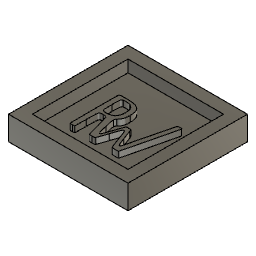
Experiment-Initials Revisited v3 (Autodesk Fusion 360 design; units mm, degrees)
Autodesk Fusion 360 part; units mm, degrees
sketch "Sketch2" plane through (0, 0, 0) normal (0, 0, 1) x (1, 0, 0)
  line L0 (0, 0) -> (100, 0)
  line L1 (100, 0) -> (100, 100)
  line L2 (100, 100) -> (0, 100)
  line L3 (0, 100) -> (0, 0)
  constraint horizontal L0
  constraint vertical L1
  constraint horizontal L2
  constraint vertical L3
  constraint coincident L0.start L3.end
extrude "Extrude3" add sketch "Sketch2" along normal blind 20
sketch "Sketch3" plane through (0, 0, 20) normal (0, 0, 1) x (-1, 0, 0)
  line L0 (0, -100) -> (0, 0)
  line L1 (0, 0) -> (-100, 0)
  line L2 (-100, 0) -> (-100, -100)
  line L3 (-100, -100) -> (0, -100)
  line L4 (-10, -10) -> (-90, -10)
  line L5 (-90, -10) -> (-90, -90)
  line L6 (-90, -90) -> (-10, -90)
  line L7 (-10, -90) -> (-10, -10)
  constraint horizontal L4
  constraint vertical L5
  constraint horizontal L6
  constraint vertical L7
extrude "Extrude4" cut sketch "Sketch3" against normal blind 10 contours L4 L5 L6 L7
sketch "Sketch4" plane through (0, 0, 10) normal (0, 0, 1) x (-1, 0, 0)
  line L0 (-10, -90) -> (-10, -10)
  line L1 (-10, -10) -> (-90, -10)
  line L2 (-90, -10) -> (-90, -90)
  line L3 (-90, -90) -> (-10, -90)
  spline S0 degree 3 poles (-75.4628, -68.295) (-73.8753, -68.1891) (-73.6636, -68.1362) (-73.5313, -67.6071) knots 0 0 0 0 1 1 1 1
  spline S1 degree 3 poles (-73.5313, -67.6071) (-72.473, -63.0562) (-68.3455, -46.4404) (-68.1338, -45.8583) knots 0 0 0 0 1 1 1 1
  spline S2 degree 3 poles (-68.1338, -45.8583) (-67.7369, -44.7471) (-64.7736, -31.8618) (-64.5355, -30.3008) knots 0 0 0 0 1 1 1 1
  spline S3 degree 3 poles (-64.5355, -30.3008) (-64.3503, -28.8456) (-64.0063, -28.8456) (-63.8211, -30.3273) knots 0 0 0 0 1 1 1 1
  spline S4 degree 3 poles (-63.8211, -30.3273) (-63.7417, -30.8829) (-62.4453, -34.6929) (-60.9371, -38.7939) knots 0 0 0 0 1 1 1 1
  line L4 (-60.9371, -38.7939) -> (-58.1855, -46.2552)
  line L5 (-58.1855, -46.2552) -> (-55.4073, -46.2552)
  line L6 (-55.4073, -46.2552) -> (-52.6028, -46.2552)
  line L7 (-52.6028, -46.2552) -> (-50.0363, -38.4764)
  spline S5 degree 3 poles (-50.0363, -38.4764) (-48.634, -34.2166) (-47.4698, -30.4596) (-47.4698, -30.1421) knots 0 0 0 0 1 1 1 1
  spline S6 degree 3 poles (-47.4698, -30.1421) (-47.4698, -29.0308) (-46.9936, -29.6129) (-46.8348, -30.9887) knots 0 0 0 0 1 1 1 1
  spline S7 degree 3 poles (-46.8348, -30.9887) (-46.729, -31.7296) (-45.9882, -35.275) (-45.1944, -38.8204) knots 0 0 0 0 1 1 1 1
  line L8 (-45.1944, -38.8204) -> (-43.7657, -45.2762)
  line L9 (-43.7657, -45.2762) -> (-44.824, -46.1758)
  spline S8 degree 3 poles (-44.824, -46.1758) (-46.3057, -47.4723) (-47.1523, -49.0333) (-47.6021, -51.4146) knots 0 0 0 0 1 1 1 1
  spline S9 degree 3 poles (-47.6021, -51.4146) (-48.0784, -53.7958) (-48.1048, -55.8066) (-47.708, -58.1614) knots 0 0 0 0 1 1 1 1
  spline S10 degree 3 poles (-47.708, -58.1614) (-47.1788, -61.5216) (-45.7765, -63.6648) (-43.263, -65.0141) knots 0 0 0 0 1 1 1 1
  spline S11 degree 3 poles (-43.263, -65.0141) (-40.8288, -66.3106) (-38.5269, -66.6281) (-31.833, -66.6281) knots 0 0 0 0 1 1 1 1
  line L10 (-31.833, -66.6281) -> (-26.0386, -66.6281)
  line L11 (-26.0386, -66.6281) -> (-26.0386, -44.8)
  line L12 (-26.0386, -44.8) -> (-26.0386, -22.9718)
  line L13 (-26.0386, -22.9718) -> (-29.2136, -22.9718)
  line L14 (-29.2136, -22.9718) -> (-32.3886, -22.9718)
  line L15 (-32.3886, -22.9718) -> (-32.3886, -33.2377)
  line L16 (-32.3886, -33.2377) -> (-32.3886, -43.4771)
  line L17 (-32.3886, -43.4771) -> (-34.6905, -43.4241)
  line L18 (-34.6905, -43.4241) -> (-36.9659, -43.3712)
  line L19 (-36.9659, -43.3712) -> (-39.7969, -33.2377)
  line L20 (-39.7969, -33.2377) -> (-42.6015, -23.1041)
  line L21 (-42.6015, -23.1041) -> (-45.803, -23.0248)
  line L22 (-45.803, -23.0248) -> (-48.978, -22.9454)
  line L23 (-48.978, -22.9454) -> (-51.6503, -30.83)
  spline S12 degree 3 poles (-51.6503, -30.83) (-53.1319, -35.1691) (-54.4019, -39.085) (-54.5078, -39.5083) knots 0 0 0 0 1 1 1 1
  spline S13 degree 3 poles (-54.5078, -39.5083) (-54.8517, -41.1752) (-54.9311, -41.3339) (-55.1692, -40.9371) knots 0 0 0 0 1 1 1 1
  spline S14 degree 3 poles (-55.1692, -40.9371) (-55.3015, -40.7254) (-55.4073, -40.355) (-55.4073, -40.0904) knots 0 0 0 0 1 1 1 1
  spline S15 degree 3 poles (-55.4073, -40.0904) (-55.4073, -39.8258) (-56.8096, -35.8835) (-58.503, -31.3062) knots 0 0 0 0 1 1 1 1
  line L24 (-58.503, -31.3062) -> (-61.5986, -22.9983)
  line L25 (-61.5986, -22.9983) -> (-65.144, -22.9189)
  spline S16 degree 3 poles (-65.144, -22.9189) (-67.1019, -22.866) (-68.7159, -22.8925) (-68.7688, -22.9718) knots 0 0 0 0 1 1 1 1
  spline S17 degree 3 poles (-68.7688, -22.9718) (-68.8482, -23.1306) (-79.749, -68.1098) (-79.749, -68.3214) knots 0 0 0 0 1 1 1 1
  spline S18 degree 3 poles (-79.749, -68.3214) (-79.749, -68.4802) (-79.0346, -68.4802) (-75.4628, -68.295) knots 0 0 0 0 1 1 1 1
  spline S19 degree 3 poles (-78.1615, -66.6546) (-78.1615, -66.0989) (-68.1603, -24.6123) (-67.9486, -24.2683) knots 0 0 0 0 1 1 1 1
  spline S20 degree 3 poles (-67.9486, -24.2683) (-67.7105, -23.8714) (-62.6569, -23.9773) (-62.3394, -24.3741) knots 0 0 0 0 1 1 1 1
  spline S21 degree 3 poles (-62.3394, -24.3741) (-62.1807, -24.5329) (-60.8048, -28.1577) (-59.2438, -32.3646) knots 0 0 0 0 1 1 1 1
  spline S22 degree 3 poles (-59.2438, -32.3646) (-56.1217, -40.8841) (-55.9894, -41.1752) (-55.3544, -41.5985) knots 0 0 0 0 1 1 1 1
  spline S23 degree 3 poles (-55.3544, -41.5985) (-54.4548, -42.1541) (-53.8992, -40.9635) (-51.3063, -33.026) knots 0 0 0 0 1 1 1 1
  spline S24 degree 3 poles (-51.3063, -33.026) (-49.904, -28.7398) (-48.5811, -24.9562) (-48.3694, -24.6123) knots 0 0 0 0 1 1 1 1
  spline S25 degree 3 poles (-48.3694, -24.6123) (-48.0255, -24.0831) (-47.7873, -24.0302) (-45.7765, -24.0302) knots 0 0 0 0 1 1 1 1
  spline S26 degree 3 poles (-45.7765, -24.0302) (-43.6069, -24.0302) (-43.554, -24.0566) (-43.2894, -24.7446) knots 0 0 0 0 1 1 1 1
  spline S27 degree 3 poles (-43.2894, -24.7446) (-43.1307, -25.1679) (-41.8871, -29.4541) (-40.5642, -34.3225) knots 0 0 0 0 1 1 1 1
  spline S28 degree 3 poles (-40.5642, -34.3225) (-39.1884, -39.2702) (-37.8919, -43.4241) (-37.6009, -43.7681) knots 0 0 0 0 1 1 1 1
  spline S29 degree 3 poles (-37.6009, -43.7681) (-37.1511, -44.3502) (-36.913, -44.4031) (-34.7963, -44.4031) knots 0 0 0 0 1 1 1 1
  spline S30 degree 3 poles (-34.7963, -44.4031) (-31.2244, -44.4031) (-31.489, -45.1968) (-31.3303, -33.7139) knots 0 0 0 0 1 1 1 1
  line L26 (-31.3303, -33.7139) -> (-31.198, -24.1625)
  line L27 (-31.198, -24.1625) -> (-29.3723, -24.0831)
  spline S31 degree 3 poles (-29.3723, -24.0831) (-28.0759, -24.0302) (-27.4673, -24.1096) (-27.3351, -24.3477) knots 0 0 0 0 1 1 1 1
  spline S32 degree 3 poles (-27.3351, -24.3477) (-27.0705, -24.7446) (-27.0176, -64.5114) (-27.2557, -65.1464) knots 0 0 0 0 1 1 1 1
  spline S33 degree 3 poles (-27.2557, -65.1464) (-27.4938, -65.755) (-36.5426, -65.755) (-39.4794, -65.1464) knots 0 0 0 0 1 1 1 1
  spline S34 degree 3 poles (-39.4794, -65.1464) (-44.7976, -64.0616) (-46.8084, -61.2835) (-46.8084, -54.9864) knots 0 0 0 0 1 1 1 1
  spline S35 degree 3 poles (-46.8084, -54.9864) (-46.7819, -50.7531) (-46.2263, -49.1391) (-43.9244, -46.705) knots 0 0 0 0 1 1 1 1
  spline S36 degree 3 poles (-43.9244, -46.705) (-43.2365, -45.9641) (-42.9719, -45.4614) (-42.9719, -44.8529) knots 0 0 0 0 1 1 1 1
  spline S37 degree 3 poles (-42.9719, -44.8529) (-42.9719, -44.3766) (-43.6598, -40.8841) (-44.533, -37.0477) knots 0 0 0 0 1 1 1 1
  spline S38 degree 3 poles (-44.533, -37.0477) (-45.7236, -31.6502) (-46.1998, -29.9568) (-46.6232, -29.5071) knots 0 0 0 0 1 1 1 1
  spline S39 degree 3 poles (-46.6232, -29.5071) (-47.1788, -28.9779) (-47.2053, -28.9779) (-47.708, -29.4277) knots 0 0 0 0 1 1 1 1
  spline S40 degree 3 poles (-47.708, -29.4277) (-48.0519, -29.7187) (-49.0573, -32.391) (-50.4067, -36.4391) knots 0 0 0 0 1 1 1 1
  spline S41 degree 3 poles (-50.4067, -36.4391) (-51.5973, -40.011) (-52.788, -43.4506) (-53.0526, -44.0856) knots 0 0 0 0 1 1 1 1
  line L28 (-53.0526, -44.0856) -> (-53.5553, -45.2233)
  line L29 (-53.5553, -45.2233) -> (-55.4603, -45.1439)
  line L30 (-55.4603, -45.1439) -> (-57.3917, -45.0646)
  line L31 (-57.3917, -45.0646) -> (-58.0267, -43.4771)
  spline S42 degree 3 poles (-58.0267, -43.4771) (-58.3707, -42.6039) (-59.6936, -39.0321) (-60.9901, -35.5396) knots 0 0 0 0 1 1 1 1
  spline S43 degree 3 poles (-60.9901, -35.5396) (-62.2865, -32.0471) (-63.5301, -29.0308) (-63.7946, -28.8721) knots 0 0 0 0 1 1 1 1
  spline S44 degree 3 poles (-63.7946, -28.8721) (-64.1386, -28.581) (-64.3238, -28.6075) (-64.7207, -28.9779) knots 0 0 0 0 1 1 1 1
  spline S45 degree 3 poles (-64.7207, -28.9779) (-65.2763, -29.4806) (-65.3821, -29.851) (-66.6521, -35.275) knots 0 0 0 0 1 1 1 1
  spline S46 degree 3 poles (-66.6521, -35.275) (-67.6311, -39.5348) (-68.6894, -43.7946) (-69.9594, -48.6364) knots 0 0 0 0 1 1 1 1
  spline S47 degree 3 poles (-69.9594, -48.6364) (-70.3828, -50.3033) (-71.5205, -54.96) (-72.4994, -58.9552) knots 0 0 0 0 1 1 1 1
  spline S48 degree 3 poles (-72.4994, -58.9552) (-73.4519, -62.9504) (-74.3515, -66.4429) (-74.4838, -66.7075) knots 0 0 0 0 1 1 1 1
  spline S49 degree 3 poles (-74.4838, -66.7075) (-74.6955, -67.0514) (-75.0923, -67.1573) (-76.4417, -67.1573) knots 0 0 0 0 1 1 1 1
  spline S50 degree 3 poles (-76.4417, -67.1573) (-77.9498, -67.1573) (-78.1615, -67.1043) (-78.1615, -66.6546) knots 0 0 0 0 1 1 1 1
  spline S51 degree 3 poles (-32.759, -63.215) (-31.4096, -62.6329) (-31.3303, -62.236) (-31.3303, -55.1981) knots 0 0 0 0 1 1 1 1
  spline S52 degree 3 poles (-31.3303, -55.1981) (-31.3303, -50.9648) (-31.4361, -48.4248) (-31.6213, -48.0279) knots 0 0 0 0 1 1 1 1
  spline S53 degree 3 poles (-31.6213, -48.0279) (-32.124, -46.9431) (-32.9178, -46.705) (-35.4842, -46.8373) knots 0 0 0 0 1 1 1 1
  spline S54 degree 3 poles (-35.4842, -46.8373) (-40.0615, -47.1018) (-42.0194, -48.7952) (-42.7338, -53.0814) knots 0 0 0 0 1 1 1 1
  spline S55 degree 3 poles (-42.7338, -53.0814) (-43.1042, -55.3039) (-42.7338, -58.3996) (-41.9401, -59.9871) knots 0 0 0 0 1 1 1 1
  spline S56 degree 3 poles (-41.9401, -59.9871) (-41.2521, -61.31) (-39.7969, -62.5535) (-38.5534, -62.8975) knots 0 0 0 0 1 1 1 1
  spline S57 degree 3 poles (-38.5534, -62.8975) (-37.1246, -63.3208) (-33.4205, -63.506) (-32.759, -63.215) knots 0 0 0 0 1 1 1 1
  spline S58 degree 3 poles (-38.2359, -61.8656) (-39.6911, -61.4687) (-40.9876, -60.1723) (-41.4109, -58.6641) knots 0 0 0 0 1 1 1 1
  spline S59 degree 3 poles (-41.4109, -58.6641) (-41.5961, -58.0291) (-41.7548, -56.3093) (-41.7548, -54.8277) knots 0 0 0 0 1 1 1 1
  spline S60 degree 3 poles (-41.7548, -54.8277) (-41.7548, -52.5523) (-41.649, -51.9966) (-41.0934, -50.8589) knots 0 0 0 0 1 1 1 1
  spline S61 degree 3 poles (-41.0934, -50.8589) (-40.0351, -48.7158) (-38.0771, -47.8427) (-34.2407, -47.8427) knots 0 0 0 0 1 1 1 1
  line L32 (-34.2407, -47.8427) -> (-32.3886, -47.8427)
  line L33 (-32.3886, -47.8427) -> (-32.3886, -55.0923)
  line L34 (-32.3886, -55.0923) -> (-32.3886, -62.3418)
  line L35 (-32.3886, -62.3418) -> (-34.7434, -62.2625)
  spline S62 degree 3 poles (-34.7434, -62.2625) (-36.0398, -62.2096) (-37.6009, -62.0243) (-38.2359, -61.8656) knots 0 0 0 0 1 1 1 1
extrude "Extrude5" add sketch "Sketch4" along normal blind 5 contours S19 S20 S21 S22 S23 S24 S25 S26 S27 S28 S29 S30 L26 L27 S31 S32 S33 S34 S35 S36 S37 S38 S39 S40 S41 L28 L29 L30 L31 S42 S43 S44 S45 S46 S47 S48 S49 S50
